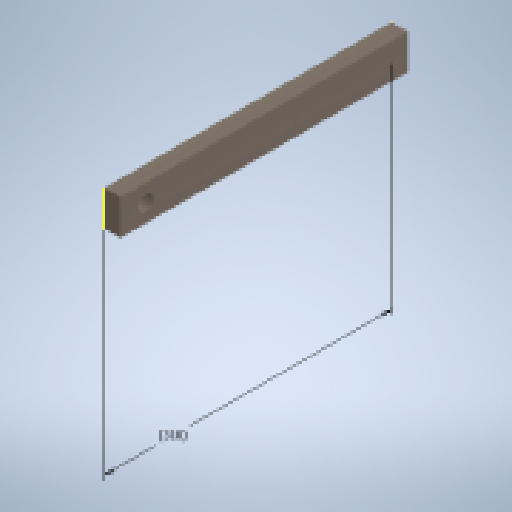
# Autodesk Inventor part: BaseUpper
Saved by Autodesk Inventor 2025.2 (Build 292293000, 293)
## iProperties
Created: 2025-03-06
Part Number: BaseUpper
Material: Wood (Walnut)
Document SubType Name: Modeling
Designer: baolo
Density: 0.55 g/cm^3
Appearance: Walnut
Mass: 92.3883 g
Surface Area: 358.032 cm^2
Volume: 167.979 cm^3
Author: baolo
Autodesk Inventor part; units mm, degrees
ref_plane "YZ Plane" through (0, 0, 0) normal (1, 0, 0) x (0, 1, 0)
ref_plane "XZ Plane" through (0, 0, 0) normal (0, 1, 0) x (-1, 0, 0)
ref_plane "XY Plane" through (0, 0, 0) normal (0, 0, 1) x (1, 0, 0)
sketch "Sketch1" plane through (0, 0, 0) normal (0, 0, 1) x (1, 0, 0)
  line L0 (7.4625, 19.05) -> (-10, 19.05)
  line L1 (-10, 19.05) -> (-10, -19.05)
  line L2 (-10, -19.05) -> (7.4625, -19.05)
  line L3 (7.4625, -19.05) -> (7.4625, 19.05)
  line L4 (-10, 135) -> (-10, -135) construction
  line L5 (0, -189) -> (0, 189) construction
  line L6 (-13.4925, 0) -> (10.955, 0) construction
  line L7 (7.4625, 19.05) -> (7.4625, 114.8156) construction
  line L8 (-10, 19.05) -> (7.4625, -19.05) construction
  line L9 (7.4625, 19.05) -> (-10, -19.05) construction
  point P0 (0, 0)
  point P1 (-1.2688, 0)
  dimension "d10" = 38.1
  constraints: 12 end point, 2 midpoint, 2 parallel, 2 point on line, 1 horizontal, 1 perpendicular
  measures "d10" distance between parallel lines of L2 L0
extrude "Extrusion1" add sketch "Sketch1" along normal blind 310
sketch "Sketch2" plane through (7.4625, -19.05, 0) normal (1, 0, 0) x (0, 0, -1)
  line L0 (17.4625, 154.05) -> (17.4625, -115.95) construction
  line L1 (-310, 0) -> (-310, 38.1) construction
  point P0 (0, 19.05)
  point P1 (-282.5375, 19.05)
  point P2 (-310, 19.05)
  dimension "d2" = 300
  constraints: 1 horizontal alignment, 1 midpoint
  measures "d2" distance from line of L0 point (-282.538, 19.05)
hole "Hole1" at (7.4625, 0, 282.5375) direction (-1, 0, 0) diameter 15.875 end through all
sketch "Sketch3" plane through (-10, -19.05, 0) normal (-1, 0, 0) x (0, 0, 1)
  line L0 (310, 38.1) -> (310, 0) projected
  line L1 (0, 38.1) -> (0, 0) projected
  point P0 (0, 19.05)
  dimension "d11" = 310
  measures "d11" distance between parallel lines of L0 L1
body "Solid1"
